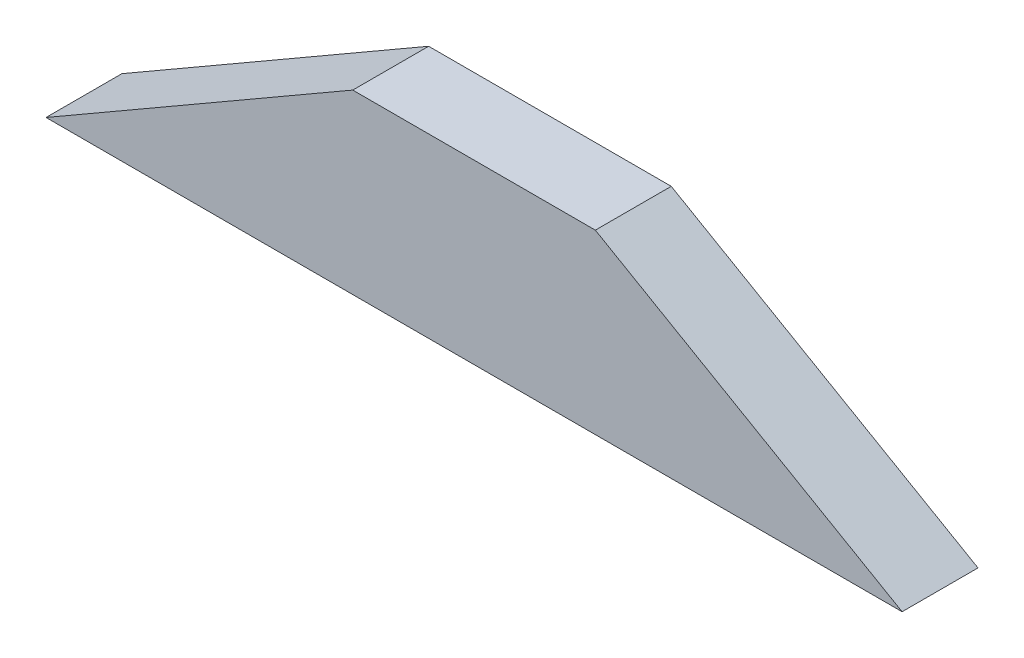
# Autodesk Inventor part: BA16
Saved by Autodesk Inventor 2017 (Build 210142000, 142)
## iProperties
Created: 2018-10-18
Part Number: BA16
Material: Wood (Oak)
Document SubType Name: Modeling
Designer: Dell
Density: 0.76 g/cm^3
Appearance: White Oak - Natural Medium Gloss
Author: Dell
Autodesk Inventor part; units mm, degrees
ref_plane "YZ Plane" through (0, 0, 0) normal (1, 0, 0) x (0, 1, 0)
ref_plane "XZ Plane" through (0, 0, 0) normal (0, 1, 0) x (-1, 0, 0)
ref_plane "XY Plane" through (0, 0, 0) normal (0, 0, 1) x (1, 0, 0)
sketch "Sketch1" plane through (0, 0, 0) normal (0, 0, 1) x (1, 0, 0)
  line L0 (0, 0) -> (429.732, 0)
  line L1 (0, 0) -> (153.9793, 88.9)
  line L2 (0, 0) -> (177.8, 0) construction
  line L3 (153.9793, 88.9) -> (275.7527, 88.9)
  line L4 (275.7527, 88.9) -> (429.732, 0)
  line L5 (153.9793, 88.9) -> (214.866, 124.053) construction
  line L6 (214.866, 124.053) -> (275.7527, 88.9) construction
  dimension "d0" = 30
  dimension "d1" = 30
  dimension "d2" = 88.9
  dimension "d3" = 248.1059
  constraints: 14 end point, 3 horizontal, 2 collinear, 1 equal length
  measures "d0" angle of L2 L1
  measures "d1" angle of L0 L4
  measures "d2" distance between parallel lines of L0 L3
  measures "d3" distance of L0.start L5.end
extrude "Extrusion1" add sketch "Sketch1" along normal blind 38.1
body "Solid1"
